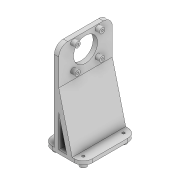
# Autodesk Inventor part: Camera_holder
Saved by Autodesk Inventor 2022 (Build 260153000, 153)
## iProperties
Created: 2022-11-09
Part Number: Camera_holder
Material: Generic
Document SubType Name: Modeling
Designer: MVeszpremi
Density: 1 g/cm^3
Appearance: Default
Author: MVeszpremi
Autodesk Inventor part; units mm, degrees
ref_plane "YZ Plane" through (0, 0, 0) normal (1, 0, 0) x (0, 1, 0)
ref_plane "XZ Plane" through (0, 0, 0) normal (0, 1, 0) x (-1, 0, 0)
ref_plane "XY Plane" through (0, 0, 0) normal (0, 0, 1) x (1, 0, 0)
sketch "Sketch1" plane through (0, 0, 0) normal (0, 1, 0) x (-1, 0, 0)
  line L0 (-15, 22.5) -> (15, 22.5)
  line L1 (15, 22.5) -> (15, -22.5)
  line L2 (15, -22.5) -> (-15, -22.5)
  line L3 (-15, -22.5) -> (-15, 22.5)
  line L4 (-15, 22.5) -> (15, -22.5) construction
  line L5 (15, 22.5) -> (-15, -22.5) construction
  circle A0 centre (15, 22.5) radius 3.5
  circle A1 centre (-15, 22.5) radius 3.5
  circle A2 centre (15, -22.5) radius 3.5
  circle A3 centre (-15, -22.5) radius 3.5
  line L6 (22.5, 30) -> (-22.5, 30)
  line L7 (-22.5, 30) -> (-22.5, -30)
  line L8 (-22.5, -30) -> (22.5, -30)
  line L9 (22.5, -30) -> (22.5, 30)
  line L10 (22.5, 30) -> (-22.5, -30) construction
  line L11 (-22.5, 30) -> (22.5, -30) construction
  circle A4 centre (15, 22.5) radius 1.45
  circle A5 centre (15, -22.5) radius 1.45
  circle A6 centre (-15, 22.5) radius 1.45
  circle A7 centre (-15, -22.5) radius 1.45
  point P0 (0, 0)
  point P1 (-11.5, 22.5)
  point P2 (-15, 19)
  point P3 (-15, -19)
  point P4 (-11.5, -22.5)
  point P5 (11.5, -22.5)
  point P6 (15, -19)
  point P7 (15, 19)
  point P8 (11.5, 22.5)
  dimension "d0" = 45
  dimension "d1" = 30
  dimension "d2" = 7
  dimension "d3" = 7
  dimension "d4" = 7
  dimension "d5" = 7
  dimension "d6" = 7.5
  dimension "d7" = 7.5
  dimension "d8" = 2.9
  dimension "d9" = 2.9
  dimension "d10" = 2.9
  dimension "d11" = 2.9
  constraints: 24 end point, 8 centre point, 7 coincident, 4 midpoint, 4 parallel, 2 horizontal, 2 perpendicular
  measures "d0" distance of L0.end L1.end
  measures "d1" distance of L0.start L0.end
  measures "d2" diameter of A0
  measures "d3" diameter of A1
  measures "d4" diameter of A2
  measures "d5" diameter of A3
  measures "d6" distance between parallel lines of L9 L1
  measures "d7" distance between parallel lines of L0 L6
  measures "d8" diameter of A4
  measures "d9" diameter of A5
  measures "d10" diameter of A6
  measures "d11" diameter of A7
extrude "Extrusion1" add sketch "Sketch1" against normal blind 5 contours A6 L3 A1 L0 | L0 A1 L3 A6 | A0 L1 A4 L0 | L0 A4 L1 A0 | A3 L2 A7 L3 | L3 A7 L2 A3 | A2 L2 A5 L1 | L1 A5 L2 A2
extrude "Extrusion2" add sketch "Sketch1" along normal blind 4 contours A6 L3 A1 L0 | L0 A1 L3 A6 | L0 A0 L1 A2 L2 A3 L3 A1 | A0 L1 A4 L0 | L0 A4 L1 A0 | A3 L2 A7 L3 | L3 A7 L2 A3 | A2 L2 A5 L1 | L1 A5 L2 A2 | L9 L8 L7 L6
sketch "Sketch2" plane through (0, 4, 0) normal (0, 1, 0) x (1, 0, 0)
  line L0 (-10, -30) -> (-5, -30)
  line L1 (-5, -30) -> (-5, 30)
  line L2 (-5, 30) -> (-10, 30)
  line L3 (-10, 30) -> (-10, -30)
  line L4 (-10, -30) -> (-5, 30) construction
  line L5 (-5, -30) -> (-10, 30) construction
  point P0 (0, 0)
  point P1 (-7.5, 0)
  dimension "d39" = 60
  dimension "d40" = 5
  dimension "d41" = 5
  constraints: 12 end point, 2 midpoint, 2 parallel, 1 horizontal, 1 perpendicular
  measures "d39" distance of L2.end L0.start
  measures "d40" distance of L0.start L0.end
  measures "d41" horizontal distance of point (0, 0) L0.end
extrude "Extrusion3" add sketch "Sketch2" along normal blind 100
sketch "Sketch3" plane through (-5, 4, 30) normal (1, 0, 0) x (0, 0, -1)
  line L0 (30, 100) -> (30, 82.5)
  line L1 (16.25, 68.75) -> (43.75, 68.75)
  line L2 (43.75, 68.75) -> (43.75, 96.25)
  line L3 (43.75, 96.25) -> (16.25, 96.25)
  line L4 (16.25, 96.25) -> (16.25, 68.75)
  line L5 (16.25, 68.75) -> (43.75, 96.25) construction
  line L6 (43.75, 68.75) -> (16.25, 96.25) construction
  circle A0 centre (16.25, 96.25) radius 1.25
  circle A1 centre (43.75, 96.25) radius 1.25
  circle A2 centre (16.25, 68.75) radius 1.25
  circle A3 centre (43.75, 68.75) radius 1.25
  circle A4 centre (30, 82.5) radius 13.5
  circle A5 centre (16.25, 96.25) radius 3
  circle A6 centre (43.75, 96.25) radius 3
  circle A7 centre (16.25, 68.75) radius 3
  circle A8 centre (43.75, 68.75) radius 3
  line L7 (0, 100) -> (60, 100) projected
  line L8 (60, 0) -> (60, 100) projected
  point P0 (30, -4)
  dimension "d19" = 27.5
  dimension "d20" = 27.5
  dimension "d21" = 2.5
  dimension "d22" = 2.5
  dimension "d23" = 2.5
  dimension "d24" = 2.5
  dimension "d26" = 27
  dimension "d27" = 6
  dimension "d28" = 6
  dimension "d29" = 6
  dimension "d30" = 6
  dimension "d42" = 17.5
  dimension "d53" = 30
  constraints: 14 end point, 9 centre point, 9 coincident, 3 midpoint, 2 parallel, 1 horizontal, 1 perpendicular, 1 vertical
  measures "d19" distance of L2.end L3.end
  measures "d20" distance of L1.end L2.end
  measures "d21" diameter of A0
  measures "d22" diameter of A1
  measures "d23" diameter of A2
  measures "d24" diameter of A3
  measures "d26" diameter of A4
  measures "d27" diameter of A5
  measures "d28" diameter of A6
  measures "d29" diameter of A7
  measures "d30" diameter of A8
  measures "d42" distance of L0.start L0.end
  measures "d53" distance between parallel lines of L8 L0
extrude "Extrusion4" cut sketch "Sketch3" against normal blind 60 contours L4 A2 L1 | L1 A2 L4 | A3 L2 L1 | L1 L2 A3 | A0 L3 L4 | L4 L3 A0 | A1 L3 L2 | L2 L3 A1 | A4
extrude "Extrusion5" add sketch "Sketch3" along normal blind 5 contours A2 L4 A7 L1 | L1 A7 L4 A2 | A8 L2 A3 L1 | L1 A3 L2 A8 | A5 L3 A0 L4 | L4 A0 L3 A5 | A6 L3 A1 L2 | L2 A1 L3 A6
fillet "Fillet1" radius 10 2 edges at (-7.5, 104, -30) (-7.5, 104, 30)
sketch "Sketch6" plane through (-10, 4, 30) normal (0, 0, 1) x (-1, 0, 0)
  line L0 (-5, 0) -> (-5, -90) projected
  line L1 (-5, -60) -> (-20, 0)
  line L2 (12.5, 0) -> (-32.5, 0) projected
  line L3 (-5, -36) -> (-14, 0)
  line L4 (-32.5, 0) -> (12.5, 0) projected
  line L5 (12.5, 4) -> (-32.5, 4) projected
  point P0 (-10, 4)
  point P1 (-10, 0)
  dimension "d50" = 40
  dimension "d52" = 15
  dimension "d54" = 60
  constraints: 4 end point, 4 point on line, 1 midpoint, 1 parallel
  measures "d50" distance from line of L5 L3.start
  measures "d52" distance of L0.start L1.end
  measures "d54" distance of L0.start L1.start
extrude "Extrusion7" add sketch "Sketch6" against normal up to surface (60 mm away) contours L0 L1 L2 L3
fillet "Fillet2" radius 10 4 edges at (22.5, 2, 30) (-22.5, 2, 30) (22.5, 2, -30) (-22.5, 2, -30)
body "Solid1"
